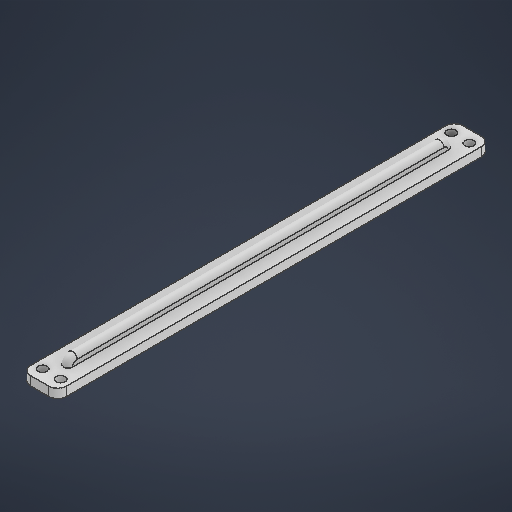
# Autodesk Inventor part: structural_bar1
Saved by Autodesk Inventor 2026.1 (Build 301233000, 233)
## iProperties
Created: 2026-05-17
Part Number: structural_bar1
Material: Generic
Document SubType Name: Modeling
Designer: emanuel
Density: 1 g/cm^3
Appearance: Default
Author: emanuel
Autodesk Inventor part; units mm, degrees
ref_plane "YZ Plane" through (0, 0, 0) normal (1, 0, 0) x (0, 1, 0)
ref_plane "XZ Plane" through (0, 0, 0) normal (0, 1, 0) x (-1, 0, 0)
ref_plane "XY Plane" through (0, 0, 0) normal (0, 0, 1) x (1, 0, 0)
sketch "Sketch1" plane through (0, 0, 0) normal (0, 1, 0) x (-1, 0, 0)
  line L0 (0, 0) -> (12, 0)
  line L1 (12, 0) -> (12, -144.6)
  line L2 (12, -144.6) -> (0, -144.6)
  line L3 (0, -144.6) -> (0, 0)
  line L4 (0, 0) -> (3, 0)
  line L5 (3, 0) -> (3, -4)
  line L6 (3, -4) -> (0, -4)
  line L7 (0, -4) -> (0, 0)
  line L8 (3, -4) -> (9, -4)
  circle A0 centre (9, -4) radius 1.5
  circle A1 centre (3, -4) radius 1.5
  line L9 (12, -144.6) -> (9, -144.6)
  line L10 (9, -144.6) -> (9, -140.6)
  line L11 (9, -140.6) -> (12, -140.6)
  line L12 (12, -140.6) -> (12, -144.6)
  line L13 (9, -140.6) -> (3, -140.6)
  circle A2 centre (9, -140.6) radius 1.5
  circle A3 centre (3, -140.6) radius 1.5
  dimension "d0" = 12
  dimension "d1" = 144.6
  dimension "d2" = 3
  dimension "d3" = 4
  dimension "d4" = 6
  dimension "d5" = 3
  dimension "d6" = 3
  dimension "d7" = 3
  dimension "d8" = 4
  dimension "d9" = 6
  dimension "d10" = 3
  dimension "d11" = 3
  constraints: 28 end point, 6 parallel, 5 horizontal, 4 centre point, 4 coincident, 3 perpendicular
  measures "d0" distance of L1.end L2.end
  measures "d1" distance of L0.end L1.end
  measures "d2" distance of L5.end L6.end
  measures "d3" distance of L4.end L5.end
  measures "d4" distance of L5.end L8.end
  measures "d5" diameter of A0
  measures "d6" diameter of A1
  measures "d7" distance of L10.end L11.end
  measures "d8" distance of L9.end L10.end
  measures "d9" distance of L10.end L13.end
  measures "d10" diameter of A2
  measures "d11" diameter of A3
extrude "Extrusion1" add sketch "Sketch1" along normal blind 3 contours L0 L5 A1 L6 L3 | L0 L1 L11 A2 L10 L2 L3 L6 A1 L5 | L1 L2 L10 A2 L11
sketch "Sketch2" plane through (0, 3, 0) normal (0, 1, 0) x (1, 0, 0)
  line L0 (-12, 0) -> (0, 0) projected
  line L1 (-6, 0) -> (-6, 144.6) construction
  line L2 (0, 144.6) -> (-12, 144.6) projected
  line L3 (-4.5, 0) -> (-4.5, 144.6)
  line L4 (-7.5, 144.6) -> (-7.5, 0)
  arc A0 (-7.5, 0) -> (-4.5, 0) centre (-6, 0) ccw
  arc A1 (-4.5, 144.6) -> (-7.5, 144.6) centre (-6, 144.6) ccw
  line L5 (0, 0) -> (0, 144.6) projected
  line L6 (-12, 0) -> (0, 0)
  line L7 (0, 0) -> (0, 8)
  line L8 (0, 8) -> (-12, 8)
  line L9 (-12, 8) -> (-12, 0)
  line L10 (-12, 144.6) -> (0, 144.6)
  line L11 (0, 144.6) -> (0, 136.6)
  line L12 (0, 136.6) -> (-12, 136.6)
  line L13 (-12, 136.6) -> (-12, 144.6)
  point P0 (-6, 72.3)
  point P1 (-4.5, 136.6)
  point P2 (-7.5, 136.6)
  point P3 (-7.5, 8)
  point P4 (-4.5, 8)
  dimension "d14" = 3
  dimension "d15" = 8
  dimension "d16" = 8
  constraints: 24 end point, 5 parallel, 4 point on circle, 4 tangent, 3 midpoint, 2 centre point, 2 horizontal, 2 perpendicular, 2 point on line
  measures "d14" diameter of A1
  measures "d15" distance of L7.end L6.end
  measures "d16" distance of L10.end L11.end
extrude "Extrusion2" add sketch "Sketch2" along normal blind 3 contours L4 L12 L3 L8
fillet "Fillet1" radius 3 2 edges at (-6, 6, -8) (-6, 6, -136.6)
fillet "Fillet2" radius 3 4 edges at (0, 1.5, 0) (-12, 1.5, 0) (-12, 1.5, -144.6) (0, 1.5, -144.6)
fillet "Fillet3" radius 1.5 10 edges at (-7.5, 3.0001, -8) (-7.5, 5.1213, -8.8787) (-7.5, 3.0001, -136.6) (-7.5, 5.1213, -135.7213) (-7.5, 6, -72.3) (-4.5, 3.0001, -136.6) (-4.5, 5.1213, -135.7213) (-4.5, 3.0001, -8) (-4.5, 5.1213, -8.8787) (-4.5, 6, -72.3)
body "Solid1"
